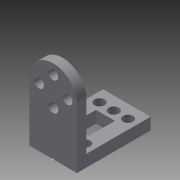
# Autodesk Inventor part: ClawJoint
Saved by Autodesk Inventor 2015 (Build 190159000, 159)
## iProperties
Created: 2016-04-24
Part Number: ClawJoint
Material: Generic
Document SubType Name: Modeling
Designer: Hatch
Density: 1 g/cm^3
Appearance: Default
Author: Hatch
Autodesk Inventor part; units mm, degrees
ref_plane "YZ Plane" through (0, 0, 0) normal (1, 0, 0) x (0, 1, 0)
ref_plane "XZ Plane" through (0, 0, 0) normal (0, 1, 0) x (-1, 0, 0)
ref_plane "XY Plane" through (0, 0, 0) normal (0, 0, 1) x (1, 0, 0)
sketch "Sketch1" plane through (0, 0, 0) normal (0, 1, 0) x (-1, 0, 0)
  circle A0 centre (0, 0) radius 10
  dimension "d0" = 20
  constraints: 1 centre point, 1 coincident
  measures "d0" diameter of A0
extrude "Extrusion1" add sketch "Sketch1" along normal blind 4
sketch "Sketch2" plane through (0, 4, 0) normal (0, 1, 0) x (1, 0, 0)
  line L0 (0, 0) -> (0, 6)
  circle A0 centre (0, 6) radius 2.125
  dimension "d3" = 6
  dimension "d4" = 4.25
  constraints: 2 end point, 1 centre point, 1 coincident, 1 vertical
  measures "d3" distance of L0.start L0.end
  measures "d4" diameter of A0
extrude "Extrusion2" cut sketch "Sketch2" against normal through all
pattern_circular "Circular Pattern1" count 4 over 360 about axis through (0, 0, 0) along (0, 1, 0) of "Extrusion2"
sketch "Sketch3" plane through (0, 0, 0) normal (0, -1, 0) x (1, 0, 0)
  circle A0 centre (0, 0) radius 10 projected
  arc A1 (-10, 0) -> (10, 0) centre (0, 0) ccw
  line L0 (10, 0) -> (10, -25)
  line L1 (10, -25) -> (-10, -25)
  line L2 (-10, -25) -> (-10, 0)
  dimension "d10" = 25
  constraints: 6 end point, 2 perpendicular, 2 point on circle, 2 tangent, 2 vertical, 1 centre point, 1 horizontal alignment, 1 other
  measures "d10" distance of L0.start L0.end
extrude "Extrusion3" add sketch "Sketch3" against normal blind 4 contours L0 L1 L2 A0
sketch "Sketch4" plane through (0, 4, 0) normal (0, 1, 0) x (1, 0, 0)
  line L0 (-10, 25) -> (-10, 0) projected
  line L1 (10, 25) -> (-10, 25)
  line L2 (-10, 25) -> (-10, 20)
  line L3 (-10, 20) -> (10, 20)
  line L4 (10, 20) -> (10, 25)
  point P0 (0, 0)
  dimension "d13" = 5
  constraints: 8 end point, 2 parallel, 1 horizontal, 1 perpendicular, 1 point on line
  measures "d13" distance of L2.end L1.end
extrude "Extrusion4" add sketch "Sketch4" along normal blind 27
sketch "Sketch5" plane through (10, 0, -25) normal (0, 0, -1) x (-1, 0, 0)
  point P0 (10, 0)
sketch "Sketch6" plane through (10, 0, -25) normal (0, 0, -1) x (-1, 0, 0)
  line L0 (7.875, 4) -> (12.125, 4) projected
  line L1 (20, 31) -> (0, 31) projected
  line L2 (10, 17.5) -> (20, 17.5)
  line L3 (10, 17.5) -> (10, 23.5)
  line L4 (10, 23.5) -> (10, 25.5)
  circle A0 centre (10, 25.5) radius 2.125
  point P0 (10, 0)
  dimension "d16" = 6
  dimension "d26" = 2
  dimension "d27" = 4.25
  constraints: 6 end point, 2 coincident, 1 centre point, 1 horizontal, 1 vertical
  measures "d16" distance of L2.start L3.end
  measures "d26" distance of L4.start L4.end
  measures "d27" diameter of A0
extrude "Extrusion5" cut sketch "Sketch6" against normal through all
pattern_linear "Rectangular Pattern1" count 3 spacing 6 along (-1, 0, 0) count 2 spacing 18 along (0, -1, 0) of "Extrusion5" first direction both ways yes
sketch "Sketch7" plane through (-10, 4, -20) normal (0, 0, 1) x (1, 0, 0)
  circle A0 centre (10, 21.5) radius 2.125 projected
  circle A1 centre (10, 3.5) radius 2.125 projected
  line L0 (10, 21.5) -> (10, 3.5)
  line L1 (6, 7) -> (14, 7)
  line L2 (14, 7) -> (14, 18)
  line L3 (14, 18) -> (6, 18)
  line L4 (6, 18) -> (6, 7)
  line L5 (6, 7) -> (14, 18) construction
  line L6 (14, 7) -> (6, 18) construction
  point P0 (10, -4)
  point P1 (10, 12.5)
  dimension "d29" = 8
  dimension "d30" = 11
  constraints: 14 end point, 3 midpoint, 2 parallel, 1 horizontal, 1 perpendicular, 1 vertical
  measures "d29" distance of L3.end L2.end
  measures "d30" distance of L2.end L1.end
extrude "Extrusion6" cut sketch "Sketch7" against normal through all contours L3 L2 L1 L0 | L0 L1 L4 L3
body "Solid1"
